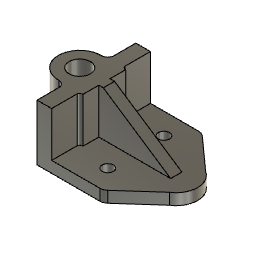
A3 (Autodesk Fusion 360 design; units mm, degrees)
Autodesk Fusion 360 part; units mm, degrees
sketch "Base_Sketch" plane through (0, 0, 0) normal (0, 0, 1) x (1, 0, 0)
  line L0 (-40, 44) -> (16.0721, 44)
  line L1 (16.0721, -44) -> (-40, -44)
  line L2 (-24, 5) -> (-24, 18.9991)
  line L3 (-24, -5) -> (-24, -18.9991)
  arc A0 (-27, 21.2952) -> (-24, 18.9991) centre (-24.0835, 21.9979) ccw
  line L4 (-27, 44) -> (-27, 21.2952)
  line L5 (-27, -21.2952) -> (-27, -44)
  arc A1 (-27, -17.4935) -> (-27, -17.4935) centre (-24.0728, -22.0228) ccw
  line L6 (-20, 0) -> (-20, 5)
  line L7 (-20, 5) -> (-20, 0)
  line L8 (-20, 0) -> (-20, -5)
  line L9 (-20, 5) -> (-24, 5)
  line L10 (-20, -5) -> (-24, -5)
  circle A2 centre (-46, 0.0012) radius 9.5
  arc A3 (-45.4349, 18.9928) -> (-45.4349, -18.9904) centre (-46, 0.0012) ccw
  arc A4 (-45.4349, 18.9928) -> (-40, 23.5243) centre (-45.8206, 24.9804) ccw
  line L11 (-40, -44) -> (-40, -23.5218)
  line L12 (-40, 23.5243) -> (-40, 44)
  arc A5 (-40, -23.5218) -> (-45.4349, -18.9904) centre (-45.8206, -24.978) ccw
  arc A6 (-24, -18.9991) -> (-27, -21.2952) centre (-24.0835, -21.9979) ccw
  arc A7 (50.0608, -16.1177) -> (50.0608, 16.1177) centre (40, 0) ccw
  circle A8 centre (4, 25) radius 5
  circle A9 centre (4, -25) radius 5
  line L13 (50.0608, -16.1177) -> (21.0769, -42.0859)
  arc A10 (16.0721, -44) -> (21.0769, -42.0859) centre (16.0721, -36.5) ccw
  line L14 (50.0608, 16.1177) -> (21.0769, 42.0859)
  arc A11 (21.0769, 42.0859) -> (16.0721, 44) centre (16.0721, 36.5) ccw
  dimension "d3" = 13
  dimension "d7" = 3
  dimension "d9" = 4
  dimension "d11" = 19
  dimension "d12" = 38
  dimension "d13" = 12
  dimension "d14" = 38
  dimension "d19" = 10
  dimension "d22" = 7.5
  constraint horizontal L0
  constraint parallel L0 L1
  constraint coincident L0 L4.start
  constraint coincident L1 L5.end
  constraint perpendicular L1 L4
  constraint vertical L2
  constraint parallel L2 L3
  constraint collinear L4 L5
  constraint coincident L5 A1.start
  constraint perpendicular L2 L9
  constraint perpendicular L3 L10
  constraint concentric A2 A3
  constraint coincident A4.end L11
  constraint collinear L11 L12
  constraint tangent L13 A10
  measures "d3" distance of L4 L11
  measures "d7" distance of L3 L4
  measures "d9" distance of L2 L7
  measures "d11" diameter of A2
  measures "d12" diameter of A3
  measures "d13" diameter of A4
  measures "d14" diameter of A7
  measures "d19" diameter of A8
  measures "d22" radius of A10
extrude "Extrude1" add sketch "Base_Sketch" along normal blind 10 contours L0 L1 L2 L3 A0 L4 L5 A1 L6 L7 L8 L9 L10 A7 L13 A10 L14 A11 | L3 L5 A1 A6 picked at (-23.8485, -22.1321)
extrude "Extrude2" add sketch "Base_Sketch" along normal blind 50 contours L0 L1 L2 L3 A0 L4 L5 A1 L6 L7 L8 L9 L10 A3 A4 L11 L12 A5 | L3 L5 A1 A6 picked at (-28.5466, -20.9909)
sketch "Triangle_Sketch" plane through (0, 0, 0) normal (0, 1, 0) x (1, 0, 0)
  line L0 (-20, -50) -> (-20, -10)
  line L1 (-20, -10) -> (40, -10)
  line L2 (40, -10) -> (-20, -50)
  dimension "d27" = 60
  constraint vertical L0
  constraint perpendicular L0 L1
  measures "d27" distance of L0.end L1.end
extrude "Extrude3" add sketch "Triangle_Sketch" along normal mid plane 10
named bodies: "A3_Body"
